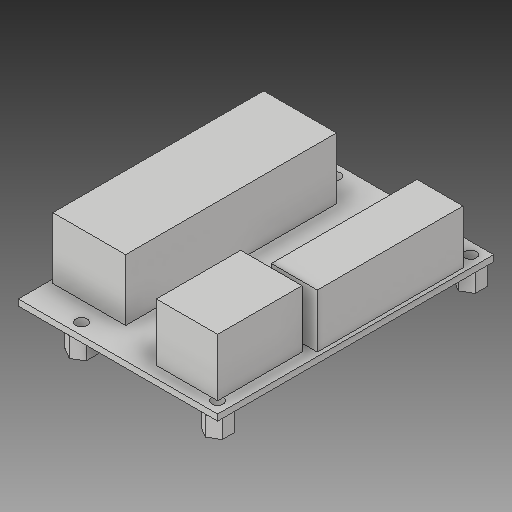
# Autodesk Inventor part: backboard
Saved by Autodesk Inventor 2018 (Build 220112000, 112)
## iProperties
Created: 2017-02-10
Part Number: backboard
Material: Generic
Document SubType Name: Modeling
Designer: steve
Density: 1 g/cm^3
Appearance: Default
Mass: 34.7117 g
Surface Area: 133.701 cm^2
Volume: 34.7117 cm^3
Vendor: Rhoban
Provider: Electronics
Author: steve
Autodesk Inventor part; units mm, degrees
ref_plane "YZ Plane" through (0, 0, 0) normal (1, 0, 0) x (0, 1, 0)
ref_plane "XZ Plane" through (0, 0, 0) normal (0, 1, 0) x (-1, 0, 0)
ref_plane "XY Plane" through (0, 0, 0) normal (0, 0, 1) x (1, 0, 0)
sketch "Sketch1" plane through (0, 0, 0) normal (0, 1, 0) x (-1, 0, 0)
  line L0 (-26, 36) -> (26, 36)
  line L1 (26, 36) -> (26, -36)
  line L2 (26, -36) -> (-26, -36)
  line L3 (-26, -36) -> (-26, 36)
  line L4 (-26, 36) -> (26, -36) construction
  line L5 (26, 36) -> (-26, -36) construction
  point P0 (0, 0)
  dimension "d0" = 72
  dimension "d1" = 52
  constraints: 12 end point, 2 midpoint, 2 parallel, 1 horizontal, 1 perpendicular
  measures "d0" distance of L0.end L1.end
  measures "d1" distance of L1.end L2.end
extrude "Extrusion1" add sketch "Sketch1" along normal blind 1.6
sketch "Sketch2" plane through (0, 1.6, 0) normal (0, 1, 0) x (1, 0, 0)
  line L0 (-12.5, -33) -> (23, -33) construction
  line L1 (23, -33) -> (23, 33) construction
  line L2 (23, 33) -> (-12.5, 33) construction
  line L3 (-12.5, 33) -> (-12.5, -33) construction
  line L4 (-12.5, -33) -> (23, 33) construction
  line L5 (23, -33) -> (-12.5, 33) construction
  line L6 (26, 36) -> (-26, 36) construction
  line L7 (-26, -36) -> (26, -36) construction
  line L8 (26, -36) -> (26, 36) construction
  line L9 (26, 36) -> (-26, 36) construction
  line L10 (-26, 36) -> (-26, -36) construction
  point P0 (0, 0)
  point P1 (5.25, 0)
  dimension "d4" = 66
  dimension "d5" = 35.5
  dimension "d6" = 3
  dimension "d7" = 3
  constraints: 12 end point, 4 coincident, 2 midpoint, 2 parallel, 1 horizontal, 1 perpendicular
  measures "d4" distance of L0.end L1.end
  measures "d5" distance of L1.end L2.end
  measures "d6" distance between parallel lines of L6 L2
  measures "d7" distance between parallel lines of L1 L8
hole "Hole1" at (-12.5, 1.6, 33) at (-12.5, 1.6, -33) at (23, 1.6, -33) at (23, 1.6, 33) direction (0, -1, 0) diameter 3 end through all
sketch "Sketch3" plane through (0, 1.6, 0) normal (0, 1, 0) x (1, 0, 0)
  line L0 (13, -9) -> (25, -9)
  line L1 (25, -9) -> (25, 29)
  line L2 (25, 29) -> (13, 29)
  line L3 (13, 29) -> (13, -9)
  circle A0 centre (23, 33) radius 1.5 construction
  line L4 (26, -36) -> (26, 36) construction
  point P0 (0, 0)
  dimension "d15" = 38
  dimension "d16" = 12
  dimension "d18" = 4
  dimension "d19" = 1
  constraints: 8 end point, 2 parallel, 1 horizontal, 1 perpendicular
  measures "d15" distance of L2.end L0.start
  measures "d16" distance of L0.start L0.end
  measures "d18" distance from line of A0.centre L2
  measures "d19" distance between parallel lines of L1 L4
extrude "Extrusion2" add sketch "Sketch3" along normal blind 14
sketch "Sketch4" plane through (0, 1.6, 0) normal (0, 1, 0) x (1, 0, 0)
  line L0 (7, -33) -> (23, -33)
  line L1 (23, -33) -> (23, -11)
  line L2 (23, -11) -> (7, -11)
  line L3 (7, -11) -> (7, -33)
  line L4 (13, -9) -> (13, 29) construction
  line L5 (13, 29) -> (25, 29) construction
  line L6 (25, 29) -> (25, -9) construction
  line L7 (25, -9) -> (13, -9) construction
  circle A0 centre (23, 33) radius 1.5 construction
  circle A1 centre (-12.5, -33) radius 1.5 construction
  circle A2 centre (-12.5, 33) radius 1.5 construction
  circle A3 centre (23, -33) radius 1.5 construction
  line L8 (-26, -36) -> (26, -36) construction
  line L9 (26, -36) -> (26, 36) construction
  line L10 (26, 36) -> (-26, 36) construction
  line L11 (-26, 36) -> (-26, -36) construction
  point P0 (0, 0)
  dimension "d22" = 22
  dimension "d23" = 16
  constraints: 8 end point, 2 parallel, 1 coincident, 1 horizontal, 1 perpendicular
  measures "d22" distance of L2.end L0.start
  measures "d23" distance of L0.start L0.end
extrude "Extrusion3" add sketch "Sketch4" along normal blind 15
sketch "Sketch5" plane through (0, 1.6, 0) normal (0, 1, 0) x (1, 0, 0)
  line L0 (-25, -28) -> (-6, -28)
  line L1 (-6, -28) -> (-6, 27)
  line L2 (-6, 27) -> (-25, 27)
  line L3 (-25, 27) -> (-25, -28)
  line L4 (-26, -36) -> (26, -36) projected
  line L5 (-26, 36) -> (-26, -36) projected
  point P0 (0, 0)
  dimension "d26" = 55
  dimension "d27" = 19
  dimension "d28" = 8
  dimension "d29" = 1
  constraints: 8 end point, 2 parallel, 1 horizontal, 1 perpendicular
  measures "d26" distance of L2.end L0.start
  measures "d27" distance of L1.end L2.end
  measures "d28" distance between parallel lines of L4 L0
  measures "d29" distance between parallel lines of L3 L5
extrude "Extrusion4" add sketch "Sketch5" along normal blind 16
sketch "Sketch6" plane through (0, 0, 0) normal (0, -1, 0) x (1, 0, 0)
  circle A0 centre (23, 33) radius 1.5 projected
  circle A1 centre (23, -33) radius 1.5 projected
  circle A2 centre (-12.5, -33) radius 1.5 projected
  circle A3 centre (-12.5, 33) radius 1.5 projected
  line L0 (25.75, 31.4123) -> (23, 29.8246)
  line L1 (23, 29.8246) -> (20.25, 31.4123)
  line L2 (20.25, 31.4123) -> (20.25, 34.5877)
  line L3 (20.25, 34.5877) -> (23, 36.1754)
  line L4 (23, 36.1754) -> (25.75, 34.5877)
  line L5 (25.75, 34.5877) -> (25.75, 31.4123)
  line L6 (20.25, -31.4123) -> (23, -29.8246)
  line L7 (23, -29.8246) -> (25.75, -31.4123)
  line L8 (25.75, -31.4123) -> (25.75, -34.5877)
  line L9 (25.75, -34.5877) -> (23, -36.1754)
  line L10 (23, -36.1754) -> (20.25, -34.5877)
  line L11 (20.25, -34.5877) -> (20.25, -31.4123)
  line L12 (-9.75, 31.4123) -> (-12.5, 29.8246)
  line L13 (-12.5, 29.8246) -> (-15.25, 31.4123)
  line L14 (-15.25, 31.4123) -> (-15.25, 34.5877)
  line L15 (-15.25, 34.5877) -> (-12.5, 36.1754)
  line L16 (-12.5, 36.1754) -> (-9.75, 34.5877)
  line L17 (-9.75, 34.5877) -> (-9.75, 31.4123)
  line L18 (-9.75, -31.4123) -> (-9.75, -34.5877)
  line L19 (-9.75, -34.5877) -> (-12.5, -36.1754)
  line L20 (-12.5, -36.1754) -> (-15.25, -34.5877)
  line L21 (-15.25, -34.5877) -> (-15.25, -31.4123)
  line L22 (-15.25, -31.4123) -> (-12.5, -29.8246)
  line L23 (-12.5, -29.8246) -> (-9.75, -31.4123)
  line L24 (26, -36) -> (26, 36) projected
  line L25 (-26, 36) -> (-26, -36) projected
  point P0 (0, 0)
  dimension "d32" = 5.5
  dimension "d33" = 5.5
  dimension "d34" = 5.5
  dimension "d35" = 5.5
  constraints: 48 end point, 4 coincident, 3 parallel, 1 point on line, 52 other
  measures "d32" distance between parallel lines of L1 L4
  measures "d33" distance between parallel lines of L8 L11
  measures "d34" distance between parallel lines of L20 L23
  measures "d35" distance between parallel lines of L13 L16
extrude "Extrusion5" add sketch "Sketch6" along normal blind 5
body "Solid1"
